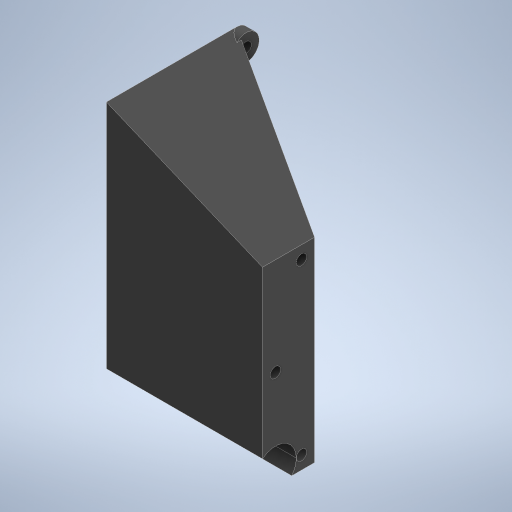
# Autodesk Inventor part: board_cover_side_right
Saved by Autodesk Inventor 2024.1 (Build 281209000, 209)
## iProperties
Created: 2024-02-15
Part Number: board_cover_side_right
Material: 一般
Document SubType Name: Modeling
Designer: hibik
Density: 1 g/cm^3
Appearance: 既定
Author: hibik
Autodesk Inventor part; units mm, degrees
ref_plane "YZ Plane" through (0, 0, 0) normal (1, 0, 0) x (0, 1, 0)
ref_plane "XZ Plane" through (0, 0, 0) normal (0, 1, 0) x (-1, 0, 0)
ref_plane "XY Plane" through (0, 0, 0) normal (0, 0, 1) x (1, 0, 0)
sketch "スケッチ2" plane through (0, 0, 0) normal (0, 1, 0) x (-1, 0, 0)
  line L0 (0, 0) -> (24, 0)
  line L1 (24, 0) -> (24, -8)
  line L2 (24, -8) -> (0, -8)
  line L3 (0, -8) -> (0, 0)
  line L4 (24, -8) -> (24, 12)
  line L5 (24, 12) -> (0, 0)
  dimension "d0" = 8
  dimension "d1" = 24
  dimension "d2" = 20
  constraints: 12 end point, 2 parallel, 1 collinear, 1 horizontal, 1 perpendicular
  measures "d0" distance of L2.end L0.start
  measures "d1" distance of L1.end L2.end
  measures "d2" distance of L1.end L4.end
extrude "押し出し1" add sketch "スケッチ2" along normal blind 40
sketch "スケッチ3" plane through (0, 0, -8) normal (0, 0, -1) x (-1, 0, 0)
  line L0 (0, 40) -> (24, 40) projected
  line L1 (24, 0) -> (24, 40) projected
  line L2 (0, 40) -> (24, 40)
  line L3 (24, 40) -> (24, 30)
  line L4 (24, 30) -> (0, 30)
  line L5 (0, 30) -> (0, 40)
  line L6 (0, 30) -> (24, 40)
  point P0 (0, 0)
  dimension "d5" = 10
  constraints: 10 end point, 2 parallel, 1 horizontal, 1 perpendicular, 1 point on line
  measures "d5" distance between parallel lines of L0 L4
extrude "押し出し2" cut sketch "スケッチ3" against normal through all contours L0 L6 L5
sketch "スケッチ4" plane through (0, 0, 0) normal (1, 0, 0) x (0, 0, -1)
  circle A0 centre (2, 28) radius 0.8 projected
  circle A1 centre (6, 15) radius 0.8 projected
  circle A2 centre (2, 2) radius 0.8 projected
  line L0 (0, 0) -> (8, 0) projected
  circle A3 centre (6, 2) radius 2
  circle A4 centre (6, 2) radius 3.2
  line L1 (8, 0) -> (8, 30) projected
  line L2 (2.8, 2) -> (2.8, 0)
  dimension "d11" = 4
  constraints: 2 end point, 2 horizontal alignment, 2 point on line, 2 tangent, 1 centre point, 1 coincident, 1 vertical, 3 other
  measures "d11" diameter of A3
extrude "押し出し3" cut sketch "スケッチ4" against normal through all contours A0 | A1 | A2 | A4 L1 A3 L0 | A4 L0 L1 | A3 | L1 L0 A3
sketch "スケッチ5" plane through (-24, 0, 12) normal (-1, 0, 0) x (0, 0, 1)
  line L0 (0, 0) -> (0, 40) projected
  circle A0 centre (0, 38) radius 2
  circle A1 centre (0, 38) radius 0.8
  point P0 (-12, 0)
  point P1 (0, 38.8)
  point P2 (0, 37.2)
  dimension "d12" = 4
  dimension "d13" = 1.6
  constraints: 1 centre point, 1 coincident, 1 point on line, 1 vertical alignment, 2 other
  measures "d13" diameter of A1
extrude "押し出し4" add sketch "スケッチ5" against normal blind 1.5 contours A0 L0 A1 | L0 A1 A0
extrude "押し出し5" cut sketch "スケッチ5" against normal through all contours A1 L0 picked at (-0.3045, 37.8004)
mirror "ミラー2" about plane through (0, 0, 0) normal (0, 0, 1) remove original yes
